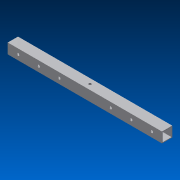
# Autodesk Inventor part: BackBottonSupport
Saved by Autodesk Inventor 2013 (Build 170138000, 138)
## iProperties
Created: 2013-07-19
Part Number: BackBottonSupport
Material: Aluminum 6061
Document SubType Name: Modeling
Designer: robotics
Density: 1 g/cm^3
Author: robotics
Autodesk Inventor part; units mm, degrees
ref_plane "YZ Plane" through (0, 0, 0) normal (1, 0, 0) x (0, 1, 0)
ref_plane "XZ Plane" through (0, 0, 0) normal (0, 1, 0) x (-1, 0, 0)
ref_plane "XY Plane" through (0, 0, 0) normal (0, 0, 1) x (1, 0, 0)
sketch "Sketch1" plane through (0, 0, 0) normal (1, 0, 0) x (0, 1, 0)
  line L0 (-10.9728, 10.9728) -> (10.9728, 10.9728)
  line L1 (10.9728, 10.9728) -> (10.9728, -10.9728)
  line L2 (10.9728, -10.9728) -> (-10.9728, -10.9728)
  line L3 (-10.9728, -10.9728) -> (-10.9728, 10.9728)
  line L4 (-10.9728, 10.9728) -> (10.9728, -10.9728) construction
  line L5 (10.9728, 10.9728) -> (-10.9728, -10.9728) construction
  line L6 (-12.7, 12.7) -> (12.7, 12.7)
  line L7 (12.7, 12.7) -> (12.7, -12.7)
  line L8 (12.7, -12.7) -> (-12.7, -12.7)
  line L9 (-12.7, -12.7) -> (-12.7, 12.7)
  line L10 (-12.7, 12.7) -> (12.7, -12.7) construction
  line L11 (12.7, 12.7) -> (-12.7, -12.7) construction
  point P0 (0, 0)
  dimension "d2" = 1.7272
  dimension "d4" = 1.7272
  dimension "d5" = 25.4
  dimension "d6" = 25.4
  constraints: 24 end point, 4 midpoint, 4 parallel, 2 horizontal, 2 perpendicular
  measures "d2" distance between parallel lines of L8 L2
  measures "d4" distance between parallel lines of L1 L7
  measures "d5" distance of L8.end L6.start
  measures "d6" distance of L6.start L6.end
extrude "Extrusion1" add sketch "Sketch1" along normal blind 381
sketch "Sketch2" plane through (0, -12.7, 12.7) normal (0, 0, 1) x (1, 0, 0)
  line L0 (0, 0) -> (0, 25.4) projected
  line L1 (381, 25.4) -> (381, 0) projected
  line L2 (0, 25.4) -> (381, 25.4) projected
  point P0 (0, 12.7)
  point P1 (25.4, 12.7)
  point P2 (355.6, 12.7)
  dimension "d9" = 25.4
  dimension "d10" = 12.7
  dimension "d11" = 25.4
  dimension "d12" = 12.7
  measures "d9" distance from line of L0 point (25.4, 12.7)
  measures "d10" distance from line of L2 point (25.4, 12.7)
  measures "d11" distance from line of point (355.6, 12.7) L1
  measures "d12" distance from line of point (355.6, 12.7) L2
hole "Hole1" at (25.4, 0, 12.7) at (355.6, 0, 12.7) direction (0, 0, -1) diameter 6.35 end through all
sketch "Sketch3" plane through (0, -12.7, 12.7) normal (0, 0, 1) x (1, 0, 0)
  line L0 (0, 0) -> (381, 0) projected
  line L1 (381, 25.4) -> (381, 0) projected
  line L2 (0, 25.4) -> (381, 25.4) projected
  line L3 (101.6, 25.4) -> (101.6, 0)
  line L4 (279.4, 25.4) -> (279.4, 0)
  line L5 (190.5, 25.4) -> (190.5, 0)
  point P0 (0, 12.7)
  point P1 (76.2, 12.7)
  point P2 (127, 12.7)
  point P3 (511.7916, 13.2861)
  point P4 (652.1971, 7.6456)
  point P5 (254, 12.7)
  point P6 (304.8, 12.7)
  dimension "d20" = 50.8
  dimension "d22" = 12.7
  dimension "d23" = 12.7
  dimension "d24" = 50.8
  dimension "d25" = 12.7
  dimension "d26" = 12.7
  dimension "d27" = 25.4
  dimension "d28" = 25.4
  dimension "d29" = 177.8
  dimension "d30" = 88.9
  dimension "d31" = 381
  dimension "d32" = 190.5
  constraints: 6 end point, 4 point on line, 2 midpoint, 2 perpendicular, 1 parallel
  measures "d20" distance of point (127, 12.7) point (76.2, 12.7)
  measures "d22" distance from line of L0 point (76.2, 12.7)
  measures "d23" distance from line of L0 point (127, 12.7)
  measures "d24" distance of point (304.8, 12.7) point (254, 12.7)
  measures "d25" distance from line of point (254, 12.7) L2
  measures "d26" distance from line of point (304.8, 12.7) L2
  measures "d27" distance from line of L3 point (76.2, 12.7)
  measures "d28" distance from line of L4 point (254, 12.7)
  measures "d29" distance between parallel lines of L3 L4
  measures "d30" distance between parallel lines of L5 L3
  measures "d31" distance of L0.start L0.end
  measures "d32" distance between parallel lines of L1 L5
hole "Hole2" at (76.2, 0, 12.7) at (127, 0, 12.7) at (511.7916, 0.5861, 12.7) at (652.1971, -5.0544, 12.7) at (254, 0, 12.7) at (304.8, 0, 12.7) direction (0, 0, -1) diameter 6.35 end through all
sketch "Sketch4" plane through (0, 12.7, 12.7) normal (0, 1, 0) x (1, 0, 0)
  line L0 (381, 25.4) -> (381, 0) projected
  line L1 (0, 25.4) -> (381, 25.4) projected
  point P0 (0, 12.7)
  point P1 (190.5, 12.7)
  dimension "d40" = 12.7
  dimension "d41" = 190.5
  measures "d40" distance from line of L1 point (190.5, 12.7)
  measures "d41" distance from line of L0 point (190.5, 12.7)
hole "Hole3" at (190.5, 12.7, 0) direction (0, -1, 0) diameter 6.35 end through all
body "Solid1"
